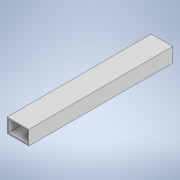
# Autodesk Inventor part: leg
Saved by Autodesk Inventor 2021 (Build 250183000, 183)
## iProperties
Created: 2022-05-07
Part Number: leg
Material: Genérico
Document SubType Name: Modeling
Designer: luzve
Density: 1 g/cm^3
Appearance: Valor por defecto
Author: luzve
Autodesk Inventor part; units mm, degrees
ref_plane "YZ Plane" through (0, 0, 0) normal (1, 0, 0) x (0, 1, 0)
ref_plane "XZ Plane" through (0, 0, 0) normal (0, 1, 0) x (-1, 0, 0)
ref_plane "XY Plane" through (0, 0, 0) normal (0, 0, 1) x (1, 0, 0)
sketch "Boceto1" plane through (0, 0, 0) normal (0, 0, 1) x (1, 0, 0)
  line L0 (0, 0) -> (60, 0)
  line L1 (60, 0) -> (60, 40)
  line L2 (60, 40) -> (0, 40)
  line L3 (0, 40) -> (0, 0)
  line L4 (3, 37) -> (57, 37)
  line L5 (57, 37) -> (57, 3)
  line L6 (57, 3) -> (3, 3)
  line L7 (3, 3) -> (3, 37)
  dimension "d0" = 60
  dimension "d1" = 40
  dimension "d2" = 3
  constraints: 16 end point, 4 parallel, 2 perpendicular, 1 horizontal, 3 other
  measures "d0" distance of L2.end L1.end
  measures "d1" distance of L1.end L0.end
  measures "d2" distance between parallel lines of L2 L4
extrude "Extrusión1" add sketch "Boceto1" along normal blind 400
